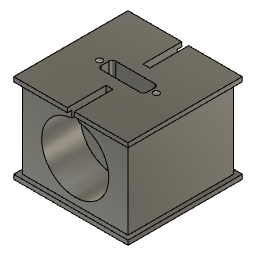
MagBody 3x1.5 V02 (Autodesk Fusion 360 design; units mm, degrees)
Autodesk Fusion 360 part; units mm, degrees
sketch "Sketch1" plane through (0, 0, 0) normal (0, 0, 1) x (1, 0, 0)
  line L0 (0, 121.92) -> (121.92, 121.92)
  line L1 (121.92, 121.92) -> (121.92, 0)
  line L2 (121.92, 0) -> (0, 0)
  line L3 (0, 0) -> (0, 121.92)
  line L4 (34.417, 69.469) -> (87.503, 69.469)
  line L5 (87.503, 69.469) -> (87.503, 52.451)
  line L6 (87.503, 52.451) -> (34.417, 52.451)
  line L7 (34.417, 52.451) -> (34.417, 69.469)
  dimension "d1" = 121.92
  dimension "d2" = 121.92
  dimension "d3" = 17.018
  dimension "d4" = 53.086
  dimension "d5" = 34.417
  dimension "d6" = 52.451
  constraint horizontal L0
  constraint vertical L1
  constraint horizontal L2
  constraint vertical L3
  constraint coincident L2.end L3.start
  constraint horizontal L4
  constraint vertical L5
  constraint horizontal L6
  constraint vertical L7
  measures "d1" distance of L0.start L0.end
  measures "d2" distance of L0.start L2.end
  measures "d3" distance of L4.end L5.end
  measures "d4" distance of L4.start L4.end
  measures "d5" distance of L3 L7
  measures "d6" distance of L2 L6
extrude "Extrude1" add sketch "Sketch1" along normal blind 102.616
sketch "Sketch2" plane through (0, 0, 0) normal (0, -1, 0) x (1, 0, 0)
  line L0 (0, 0) -> (121.92, 0)
  line L1 (121.92, 0) -> (121.92, 102.616)
  line L2 (121.92, 102.616) -> (0, 102.616)
  line L3 (0, 102.616) -> (0, 0)
  line L4 (-5.08, 102.616) -> (127, 102.616)
  line L5 (127, 102.616) -> (127, 97.536)
  line L6 (127, 97.536) -> (-5.08, 97.536)
  line L7 (-5.08, 97.536) -> (-5.08, 102.616)
  line L8 (-5.08, 0) -> (127, 0)
  line L9 (127, 0) -> (127, 5.08)
  line L10 (127, 5.08) -> (-5.08, 5.08)
  line L11 (-5.08, 5.08) -> (-5.08, 0)
  dimension "d9" = 5.08
  dimension "d10" = 132.08
  dimension "d11" = 5.08
  dimension "d12" = 132.08
  dimension "d13" = 5.08
  dimension "d14" = 5.08
  constraint horizontal L4
  constraint vertical L5
  constraint horizontal L6
  constraint vertical L7
  constraint coincident L2 L4.end
  constraint horizontal L8
  constraint vertical L9
  constraint horizontal L10
  constraint vertical L11
  constraint coincident L0.end L8
  measures "d9" distance of L4.end L5.end
  measures "d10" distance of L4.start L4.end
  measures "d11" distance of L3 L7
  measures "d12" distance of L8.start L8.end
  measures "d13" distance of L3 L11
  measures "d14" distance of L8.start L10.end
extrude "Extrude2" add sketch "Sketch2" along normal blind 5.08 contours L0 L1 L3 L8 L10 | L3 L8 L10 L11 | L1 L8 L9 L10 | L3 L4 L6 L7 | L1 L2 L3 L4 L6 | L1 L4 L5 L6
sketch "Sketch3" plane through (121.92, 0, 0) normal (1, 0, 0) x (0, 1, 0)
  line L0 (0, 0) -> (121.92, 0)
  line L1 (121.92, 0) -> (121.92, 102.616)
  line L2 (121.92, 102.616) -> (0, 102.616)
  line L3 (0, 102.616) -> (0, 97.536)
  line L4 (0, 97.536) -> (0, 5.08)
  line L5 (0, 5.08) -> (0, 0)
  line L6 (0, 102.616) -> (121.92, 102.616)
  line L7 (121.92, 102.616) -> (121.92, 97.536)
  line L8 (121.92, 97.536) -> (0, 97.536)
  line L9 (0, 97.536) -> (0, 102.616)
  line L10 (0, 0) -> (121.92, 0)
  line L11 (121.92, 0) -> (121.92, 5.08)
  line L12 (121.92, 5.08) -> (0, 5.08)
  line L13 (0, 5.08) -> (0, 0)
  dimension "d17" = 5.08
  dimension "d18" = 5.08
  constraint horizontal L6
  constraint vertical L7
  constraint horizontal L8
  constraint vertical L9
  constraint coincident L1 L7.end
  constraint coincident L2.end L3.start
  constraint horizontal L10
  constraint vertical L11
  constraint horizontal L12
  constraint vertical L13
  constraint coincident L1 L11.end
  constraint coincident L0.start L5.end
  measures "d17" distance of L1.end L7.end
  measures "d18" distance of L0.end L11.end
extrude "Extrude3" add sketch "Sketch3" along normal blind 5.08 contours L0 L1 L5 L10 L11 L12 L13 | L1 L2 L3 L6 L7 L8 L9
sketch "Sketch4" plane through (0, 121.92, 0) normal (0, 1, 0) x (-1, 0, 0)
  line L0 (-127, 0) -> (0, 0)
  line L1 (0, 0) -> (0, 102.616)
  line L2 (0, 102.616) -> (-127, 102.616)
  line L3 (-127, 102.616) -> (-127, 97.536)
  line L4 (-127, 97.536) -> (-121.92, 97.536)
  line L5 (-121.92, 97.536) -> (-121.92, 5.08)
  line L6 (-121.92, 5.08) -> (-127, 5.08)
  line L7 (-127, 5.08) -> (-127, 0)
  line L8 (-127, 102.616) -> (5.08, 102.616)
  line L9 (5.08, 102.616) -> (5.08, 97.536)
  line L10 (5.08, 97.536) -> (-127, 97.536)
  line L11 (-127, 97.536) -> (-127, 102.616)
  line L12 (-127, 5.08) -> (5.08, 5.08)
  line L13 (5.08, 5.08) -> (5.08, 0)
  line L14 (5.08, 0) -> (-127, 0)
  line L15 (-127, 0) -> (-127, 5.08)
  dimension "d21" = 5.08
  dimension "d22" = 132.08
  dimension "d23" = 132.08
  dimension "d24" = 5.08
  constraint horizontal L8
  constraint vertical L9
  constraint horizontal L10
  constraint vertical L11
  constraint coincident L2.end L3.start
  constraint horizontal L12
  constraint vertical L13
  constraint horizontal L14
  constraint vertical L15
  constraint coincident L6.end L7.start
  measures "d21" distance of L8.end L9.end
  measures "d22" distance of L2.end L8.end
  measures "d23" distance of L6.end L12.end
  measures "d24" distance of L12.end L13.end
extrude "Extrude4" add sketch "Sketch4" along normal blind 5.08 contours L0 L1 L6 L7 L12 L14 L15 | L1 L12 L13 L14 | L1 L2 L3 L4 L8 L10 L11 | L1 L8 L9 L10
sketch "Sketch5" plane through (0, 0, 0) normal (-1, 0, 0) x (0, -1, 0)
  line L0 (-121.92, 0) -> (0, 0)
  line L1 (0, 0) -> (0, 5.08)
  line L2 (0, 5.08) -> (0, 97.536)
  line L3 (0, 97.536) -> (0, 102.616)
  line L4 (0, 102.616) -> (-121.92, 102.616)
  line L5 (-121.92, 102.616) -> (-121.92, 97.536)
  line L6 (-121.92, 97.536) -> (-121.92, 5.08)
  line L7 (-121.92, 5.08) -> (-121.92, 0)
  line L8 (-121.92, 102.616) -> (0, 102.616)
  line L9 (0, 102.616) -> (0, 97.536)
  line L10 (0, 97.536) -> (-121.92, 97.536)
  line L11 (-121.92, 97.536) -> (-121.92, 102.616)
  line L12 (-121.92, 5.08) -> (0, 5.08)
  line L13 (0, 5.08) -> (0, 0)
  line L14 (0, 0) -> (-121.92, 0)
  line L15 (-121.92, 0) -> (-121.92, 5.08)
  dimension "d27" = 5.08
  dimension "d28" = 5.08
  constraint horizontal L8
  constraint vertical L9
  constraint horizontal L10
  constraint vertical L11
  constraint coincident L2.end L3.start
  constraint coincident L4.end L5.start
  constraint horizontal L12
  constraint vertical L13
  constraint horizontal L14
  constraint vertical L15
  constraint coincident L0.end L1.start
  constraint coincident L6.end L7.start
  measures "d27" distance of L4.end L5.end
  measures "d28" distance of L6.end L0.start
extrude "Extrude5" add sketch "Sketch5" along normal blind 5.08 contours L0 L1 L7 L12 L13 L14 L15 | L3 L4 L5 L8 L9 L10 L11
sketch "Sketch6" plane through (0, 0, 0) normal (0, -1, 0) x (1, 0, 0)
  line L0 (0, 5.08) -> (121.92, 5.08)
  line L1 (121.92, 5.08) -> (121.92, 97.536)
  line L2 (121.92, 97.536) -> (0, 97.536)
  line L3 (0, 97.536) -> (0, 5.08)
  circle A0 centre (60.96, 51.308) radius 38.735
  line L4 (127, 102.616) -> (-5.08, 102.616)
  dimension "d31" = 77.47
  dimension "d32" = 51.308
  dimension "d33" = 60.96
  measures "d31" diameter of A0
  measures "d32" distance of A0.centre L4
  measures "d33" distance of L3 A0.centre
extrude "Extrude6" cut sketch "Sketch6" against normal blind 44.704 contours A0
ref_plane "WorkPlane1" through (0, 60.96, 0) normal (0, 1, 0) x (0, 0, 1)
mirror "Mirror1" about plane through (0, 60.96, 0) normal (0, 1, 0) of "Extrude6"
sketch "Sketch7" plane through (0, 0, 102.616) normal (0, 0, 1) x (-1, 0, 0)
  line L0 (-87.503, -52.451) -> (-34.417, -52.451)
  line L1 (-34.417, -52.451) -> (-34.417, -69.469)
  line L2 (-34.417, -69.469) -> (-87.503, -69.469)
  line L3 (-87.503, -69.469) -> (-87.503, -52.451)
  line L4 (5.08, -127) -> (5.08, 5.08)
  line L5 (5.08, 5.08) -> (-127, 5.08)
  line L6 (-127, 5.08) -> (-127, -127)
  line L7 (-127, -127) -> (5.08, -127)
  line L8 (-57.023, -127) -> (-64.897, -127)
  line L9 (-64.897, -127) -> (-64.897, -82.296)
  line L10 (-64.897, -82.296) -> (-57.023, -82.296)
  line L11 (-57.023, -82.296) -> (-57.023, -127)
  line L12 (-33.7438, -60.96) -> (-1.1636, -60.96)
  line L13 (-64.897, -39.624) -> (-57.023, -39.624)
  line L14 (-57.023, -39.624) -> (-57.023, 5.08)
  line L15 (-64.897, 5.08) -> (-64.897, -39.624)
  line L16 (-57.023, 5.08) -> (-64.897, 5.08)
  dimension "d39" = 7.874
  dimension "d40" = 62.103
  dimension "d41" = 44.704
  constraint horizontal L8
  constraint vertical L9
  constraint horizontal L10
  constraint vertical L11
  constraint coincident L7 L8.start
  constraint symmetric L8.start L12 L14.end
  constraint symmetric L8.end L12 L15.start
  constraint symmetric L9.end L12 L13.start
  constraint symmetric L10.end L12 L13.end
  measures "d39" distance of L8.start L8.end
  measures "d40" distance of L4 L11
  measures "d41" distance of L8.start L10.end
extrude "Extrude7" cut sketch "Sketch7" against normal blind 15.24 contours L7 L8 L9 L10 L11 | L5 L13 L14 L15 L16
sketch "Sketch8" plane through (0, 0, 102.616) normal (0, 0, 1) x (-1, 0, 0)
  line L0 (-87.503, -52.451) -> (-34.417, -52.451)
  line L1 (-34.417, -52.451) -> (-34.417, -69.469)
  line L2 (-34.417, -69.469) -> (-87.503, -69.469)
  line L3 (-87.503, -69.469) -> (-87.503, -52.451)
  line L4 (-64.897, -127) -> (-64.897, -82.296)
  line L5 (-64.897, -82.296) -> (-57.023, -82.296)
  line L6 (-57.023, -82.296) -> (-57.023, -127)
  line L7 (-57.023, -127) -> (5.08, -127)
  line L8 (5.08, -127) -> (5.08, 5.08)
  line L9 (5.08, 5.08) -> (-57.023, 5.08)
  line L10 (-57.023, 5.08) -> (-57.023, -39.624)
  line L11 (-57.023, -39.624) -> (-64.897, -39.624)
  line L12 (-64.897, -39.624) -> (-64.897, 5.08)
  line L13 (-64.897, 5.08) -> (-127, 5.08)
  line L14 (-127, 5.08) -> (-127, -127)
  line L15 (-127, -127) -> (-64.897, -127)
  circle A0 centre (-28.194, -60.96) radius 4.064
  circle A1 centre (-93.726, -60.96) radius 4.064
  dimension "d44" = 8.128
  dimension "d45" = 8.128
  dimension "d46" = 33.274
  dimension "d47" = 98.806
  dimension "d48" = 66.04
  dimension "d49" = 66.04
  measures "d44" diameter of A0
  measures "d45" diameter of A1
  measures "d46" distance of L8 A0.centre
  measures "d47" distance of L8 A1.centre
  measures "d48" distance of L13 A1.centre
  measures "d49" distance of L9 A0.centre
extrude "Extrude8" cut sketch "Sketch8" against normal blind 12.7 contours A0 | A1
thread "Thread1" "ANSI Metric M Profile 8.0 M8x1.25 6H" major diameter 8.17 minor diameter 6.7795 pitch 1.25 angle 60 resizes the face on face at (24.1502, 61.3646, 94.1493)
thread "Thread2" "ANSI Metric M Profile 8.0 M8x1.25 6H" major diameter 8.17 minor diameter 6.7795 pitch 1.25 angle 60 resizes the face on face at (89.6822, 61.3646, 94.1493)
fillet "Fillet1" radius 3.81 4 edges at (87.503, 69.469, 51.308) (34.417, 69.469, 51.308) (34.417, 52.451, 51.308) (87.503, 52.451, 51.308)
